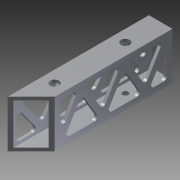
# Autodesk Inventor part: 5in 1by2 frame
Saved by Autodesk Inventor 2012 (Build 160160000, 160)
## iProperties
Created: 2013-01-04
Part Number: 5in 1by2 frame
Material: Default
Document SubType Name: Modeling
Designer: Bryce
Density: 1 g/cm^3
Author: Bryce
Autodesk Inventor part; units mm, degrees
ref_plane "YZ Plane" through (0, 0, 0) normal (1, 0, 0) x (0, 1, 0)
ref_plane "XZ Plane" through (0, 0, 0) normal (0, 1, 0) x (-1, 0, 0)
ref_plane "XY Plane" through (0, 0, 0) normal (0, 0, 1) x (1, 0, 0)
sketch "Sketch1" plane through (0, 0, 0) normal (0, 0, 1) x (1, 0, 0)
  line L0 (0, 0) -> (25.4, 0)
  line L1 (25.4, 0) -> (25.4, 50.8)
  line L2 (25.4, 50.8) -> (0, 50.8)
  line L3 (0, 50.8) -> (0, 0)
  line L4 (3.175, 3.175) -> (22.225, 3.175)
  line L5 (22.225, 3.175) -> (22.225, 47.625)
  line L6 (22.225, 47.625) -> (3.175, 47.625)
  line L7 (3.175, 47.625) -> (3.175, 3.175)
  dimension "d0" = 50.8
  dimension "d1" = 25.4
  dimension "d2" = 3.175
  dimension "d3" = 3.175
  dimension "d4" = 3.175
  dimension "d5" = 3.175
  constraints: 16 end point, 4 parallel, 2 horizontal, 2 perpendicular
  measures "d0" distance of L0.end L1.end
  measures "d1" distance of L1.end L2.end
  measures "d2" distance between parallel lines of L6 L2
  measures "d3" distance between parallel lines of L1 L5
  measures "d4" distance between parallel lines of L0 L4
  measures "d5" distance between parallel lines of L3 L7
extrude "Extrusion1" add sketch "Sketch1" along normal blind 152.4
sketch "Sketch2" plane through (0, 0, 0) normal (0, -1, 0) x (1, 0, 0)
  line L0 (25.4, 152.4) -> (0, 152.4) projected
  line L1 (0, 0) -> (0, 152.4) projected
  line L2 (25.4, 0) -> (25.4, 152.4) projected
  line L3 (0, 152.4) -> (25.4, 127)
  circle A0 centre (12.7, 114.3) radius 3.175
  circle A1 centre (12.7, 38.1) radius 3.175
  dimension "d8" = 45
  dimension "d9" = 6.35
  dimension "d10" = 12.7
  dimension "d11" = 38.1
  dimension "d12" = 76.2
  constraints: 2 centre point, 2 end point, 1 equal radius, 1 point on line, 1 vertical alignment
  measures "d8" angle of L3 L0
  measures "d9" diameter of A0
  measures "d10" distance from line of L1 A0.centre
  measures "d11" distance from line of L0 A0.centre
  measures "d12" distance of A1.centre A0.centre
extrude "Extrusion2" cut sketch "Sketch2" against normal blind 3.175 contours A0 | A1
extrude "Extrusion3" cut sketch "Sketch2" against normal through all contours L2 L3 L0
sketch "Sketch3" plane through (0, 50.8, 0) normal (0, 1, 0) x (1, 0, 0)
  circle A0 centre (12.7, -114.3) radius 3.175 projected
  circle A1 centre (12.7, -38.1) radius 3.175 projected
  circle A2 centre (12.7, -38.1) radius 4.7625
  circle A3 centre (12.7, -114.3) radius 4.7625
  dimension "d17" = 9.525
  constraints: 2 centre point, 2 coincident, 1 equal radius
  measures "d17" diameter of A2
extrude "Extrusion4" cut sketch "Sketch3" against normal blind 3.175 contours A0 | A1 | A2 | A3
sketch "Sketch4" plane through (25.4, 0, 0) normal (1, 0, 0) x (0, 0, -1)
  line L0 (-127, 50.8) -> (-127, 0) projected
  line L1 (0, 0) -> (-127, 0) projected
  line L2 (0, 0) -> (0, 50.8) projected
  line L3 (0, 50.8) -> (-127, 50.8) projected
  line L4 (0, 50.8) -> (0, 0)
  line L5 (-127, 50.8) -> (0, 50.8)
  line L6 (-127, 0) -> (-127, 50.8)
  line L7 (-127, 0) -> (0, 0)
  line L8 (-55.7727, 44.45) -> (-74.93, 12.5211)
  line L9 (-74.93, 6.35) -> (-52.07, 44.45) construction
  line L10 (-120.65, 6.35) -> (-6.35, 6.35)
  line L11 (-6.35, 44.45) -> (-120.65, 44.45)
  line L12 (-52.07, 38.2789) -> (-71.2273, 6.35)
  line L13 (-52.07, 44.45) -> (-29.21, 6.35) construction
  line L14 (-48.3673, 44.45) -> (-29.21, 12.5211)
  line L15 (-94.0873, 44.45) -> (-74.93, 12.5211)
  line L16 (-97.79, 44.45) -> (-74.93, 6.35) construction
  line L17 (-78.6327, 6.35) -> (-97.79, 38.2789)
  line L18 (-52.07, 38.2789) -> (-32.9127, 6.35)
  line L19 (-116.9473, 6.35) -> (-97.79, 38.2789)
  line L20 (-120.65, 44.45) -> (-120.65, 6.35)
  line L21 (-120.65, 6.35) -> (-97.79, 44.45) construction
  line L22 (-120.65, 12.5211) -> (-101.4927, 44.45)
  line L23 (-29.21, 12.5211) -> (-10.0527, 44.45)
  line L24 (-25.5073, 6.35) -> (-6.35, 38.2789)
  line L25 (-6.35, 6.35) -> (-6.35, 44.45)
  line L26 (-29.21, 6.35) -> (-6.35, 44.45) construction
  dimension "d20" = 30.964
  dimension "d21" = 61.928
  dimension "d22" = 61.928
  dimension "d23" = 61.928
  dimension "d24" = 61.928
  dimension "d25" = 3.175
  dimension "d26" = 3.175
  dimension "d27" = 3.175
  dimension "d28" = 3.175
  dimension "d29" = 3.175
  dimension "d30" = 3.175
  dimension "d31" = 3.175
  dimension "d32" = 3.175
  dimension "d33" = 3.175
  dimension "d34" = 3.175
  dimension "d35" = 6.35
  dimension "d36" = 6.35
  dimension "d37" = 6.35
  dimension "d38" = 6.35
  constraints: 42 end point, 8 parallel, 4 collinear, 2 point on line, 1 vertical, 20 other
  measures "d20" angle of L21 L20
  measures "d21" angle of L16 L21
  measures "d22" angle of L9 L16
  measures "d23" angle of L13 L9
  measures "d24" angle of L26 L13
  measures "d25" distance between parallel lines of L21 L22
  measures "d26" distance between parallel lines of L21 L19
  measures "d27" distance between parallel lines of L16 L17
  measures "d28" distance between parallel lines of L15 L16
  measures "d29" distance between parallel lines of L9 L8
  measures "d30" distance between parallel lines of L9 L12
  measures "d31" distance between parallel lines of L13 L18
  measures "d32" distance between parallel lines of L13 L14
  measures "d33" distance between parallel lines of L26 L23
  measures "d34" distance between parallel lines of L24 L26
  measures "d35" distance between parallel lines of L4 L25
  measures "d38" distance between parallel lines of L6 L20
extrude "Extrusion5" cut sketch "Sketch4" against normal blind 3.175 contours L8 L15 L11 | L11 L23 L14 | L22 L20 L11 | L25 L10 L24 | L19 L17 L10 | L10 L12 L18
sketch "Sketch5" plane through (0, 0, 0) normal (-1, 0, 0) x (0, 0, 1)
  line L0 (152.4, 0) -> (152.4, 50.8) projected
  line L1 (0, 50.8) -> (152.4, 50.8) projected
  line L2 (0, 50.8) -> (0, 0) projected
  line L3 (0, 0) -> (152.4, 0) projected
  line L4 (0, 0) -> (0, 50.8)
  line L5 (152.4, 0) -> (0, 0)
  line L6 (152.4, 50.8) -> (152.4, 0)
  line L7 (152.4, 50.8) -> (0, 50.8)
  line L8 (90.17, 39.0811) -> (66.1672, 6.35)
  line L9 (86.2328, 44.45) -> (62.23, 11.7189)
  line L10 (62.23, 6.35) -> (90.17, 44.45) construction
  line L11 (6.35, 6.35) -> (146.05, 6.35)
  line L12 (146.05, 44.45) -> (6.35, 44.45)
  line L13 (90.17, 44.45) -> (118.11, 6.35) construction
  line L14 (90.17, 39.0811) -> (114.1728, 6.35)
  line L15 (118.11, 11.7189) -> (142.1128, 44.45)
  line L16 (118.11, 6.35) -> (146.05, 44.45) construction
  line L17 (146.05, 6.35) -> (146.05, 44.45)
  line L18 (122.0472, 6.35) -> (146.05, 39.0811)
  line L19 (94.1072, 44.45) -> (118.11, 11.7189)
  line L20 (38.2272, 44.45) -> (62.23, 11.7189)
  line L21 (34.29, 44.45) -> (62.23, 6.35) construction
  line L22 (10.2872, 6.35) -> (34.29, 39.0811)
  line L23 (6.35, 44.45) -> (6.35, 6.35)
  line L24 (6.35, 6.35) -> (34.29, 44.45) construction
  line L25 (6.35, 11.7189) -> (30.3528, 44.45)
  line L26 (58.2928, 6.35) -> (34.29, 39.0811)
  dimension "d41" = 36.254
  dimension "d42" = 72.508
  dimension "d43" = 72.508
  dimension "d44" = 72.508
  dimension "d45" = 72.508
  dimension "d46" = 3.175
  dimension "d47" = 3.175
  dimension "d48" = 3.175
  dimension "d49" = 3.175
  dimension "d50" = 3.175
  dimension "d51" = 3.175
  dimension "d52" = 3.175
  dimension "d53" = 3.175
  dimension "d54" = 3.175
  dimension "d55" = 3.175
  dimension "d56" = 6.35
  dimension "d57" = 6.35
  dimension "d58" = 6.35
  dimension "d59" = 6.35
  constraints: 42 end point, 8 parallel, 4 collinear, 2 point on line, 1 vertical, 20 other
  measures "d41" angle of L24 L23
  measures "d42" angle of L21 L24
  measures "d43" angle of L10 L21
  measures "d44" angle of L13 L10
  measures "d45" angle of L16 L13
  measures "d46" distance between parallel lines of L24 L25
  measures "d47" distance between parallel lines of L24 L22
  measures "d48" distance between parallel lines of L21 L26
  measures "d49" distance between parallel lines of L20 L21
  measures "d50" distance between parallel lines of L10 L9
  measures "d51" distance between parallel lines of L10 L8
  measures "d52" distance between parallel lines of L13 L14
  measures "d53" distance between parallel lines of L13 L19
  measures "d54" distance between parallel lines of L16 L15
  measures "d55" distance between parallel lines of L18 L16
  measures "d56" distance between parallel lines of L4 L23
  measures "d58" distance between parallel lines of L6 L17
extrude "Extrusion6" cut sketch "Sketch5" against normal blind 3.175 contours L14 L11 L8 | L11 L22 L26 | L18 L17 L11 | L23 L12 L25 | L15 L19 L12 | L12 L9 L20
fillet "Fillet1" radius 3.175 36 edges at (1.5875, 11.7189, 6.35) (1.5875, 44.45, 6.35) (1.5875, 44.45, 30.3528) (1.5875, 39.0811, 34.29) (1.5875, 6.35, 10.2872) (1.5875, 6.35, 58.2928) (1.5875, 44.45, 38.2272) (1.5875, 11.7189, 62.23) (1.5875, 44.45, 86.2328) (1.5875, 39.0811, 90.17) (1.5875, 6.35, 66.1672) (1.5875, 6.35, 114.1728) (1.5875, 44.45, 94.1072) (1.5875, 44.45, 142.1128) (1.5875, 11.7189, 118.11) (1.5875, 39.0811, 146.05) (1.5875, 6.35, 122.0472) (1.5875, 6.35, 146.05) (23.8125, 44.45, 120.65) (23.8125, 44.45, 101.4927) (23.8125, 12.5211, 120.65) (23.8125, 6.35, 116.9473) (23.8125, 38.2789, 97.79) (23.8125, 6.35, 78.6327) (23.8125, 12.5211, 74.93) (23.8125, 44.45, 94.0873) (23.8125, 44.45, 55.7727) (23.8125, 38.2789, 52.07) (23.8125, 6.35, 71.2273) (23.8125, 6.35, 32.9127) (23.8125, 12.5211, 29.21) (23.8125, 44.45, 48.3673) (23.8125, 44.45, 10.0527) (23.8125, 38.2789, 6.35) (23.8125, 6.35, 25.5073) (23.8125, 6.35, 6.35)
equation "\"d3\" = d2"
equation "\"d4\" = d3"
equation "\"d5\" = d4"
equation "\"d21\" = 2 * d20"
equation "\"d22\" = d21"
equation "\"d23\" = d22"
equation "\"d24\" = d23"
equation "\"d26\" = d25"
equation "\"d27\" = d26"
equation "\"d28\" = d27"
equation "\"d29\" = d28"
equation "\"d30\" = d29"
equation "\"d31\" = d30"
equation "\"d32\" = d30"
equation "\"d33\" = d32"
equation "\"d34\" = d33"
equation "\"d42\" = 2 * d41"
equation "\"d43\" = d42"
equation "\"d44\" = d43"
equation "\"d45\" = d44"
equation "\"d47\" = d46"
equation "\"d48\" = d47"
equation "\"d49\" = d48"
equation "\"d50\" = d49"
equation "\"d51\" = d50"
equation "\"d52\" = d51"
equation "\"d53\" = d51"
equation "\"d54\" = d53"
equation "\"d55\" = d54"
body "Solid1"
